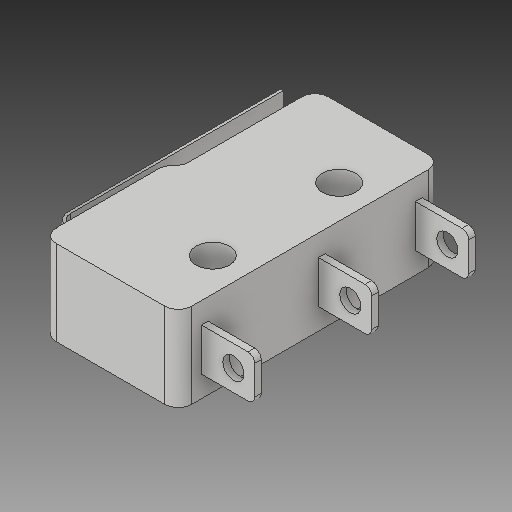
# Autodesk Inventor part: endstop_maszyna
Saved by Autodesk Inventor 2019 (Build 230136000, 136)
## iProperties
Created: 2021-11-16
Part Number: endstop_maszyna
Material: Generic
Document SubType Name: Modeling
Designer: Pokick
Density: 1 g/cm^3
Appearance: Default
Author: Pokick
Autodesk Inventor part; units mm, degrees
ref_plane "YZ Plane" through (0, 0, 0) normal (1, 0, 0) x (0, 1, 0)
ref_plane "XZ Plane" through (0, 0, 0) normal (0, 1, 0) x (-1, 0, 0)
ref_plane "XY Plane" through (0, 0, 0) normal (0, 0, 1) x (1, 0, 0)
sketch "Sketch1" plane through (0, 0, 0) normal (0, 1, 0) x (-1, 0, 0)
  line L0 (-5.1, 9.9) -> (5.1, 9.9)
  line L1 (5.1, 9.9) -> (5.1, 0.75)
  line L2 (5.1, -9.9) -> (4.4, -9.9) construction
  line L3 (-5.1, -9.9) -> (-5.1, 9.9)
  line L4 (-5.1, 9.9) -> (5.1, -9.9) construction
  line L5 (5.1, 9.9) -> (-5.1, -9.9) construction
  line L6 (0, 9.9) -> (0, 4.8) construction
  line L7 (0, 9.9) -> (5.1, 9.9) construction
  line L8 (-5.1, 4.8) -> (-2.6, 4.8) construction
  circle A0 centre (-2.6, 4.8) radius 1.25
  line L9 (-2.6, 4.8) -> (-2.6, -4.7) construction
  line L10 (-2.6, 4.8) -> (6.9, 4.8) construction
  circle A1 centre (-2.6, -4.7) radius 1.25
  line L11 (-5.1, -9.9) -> (4.4, -9.9) construction
  line L12 (-5.1, -9.9) -> (4.4, -9.9) construction
  line L13 (4.4, -9.9) -> (4.4, 0.05)
  line L14 (4.4, 0.05) -> (5.1, 0.75)
  line L15 (5.1, 0.75) -> (5.1, -9.9) construction
  line L16 (4.4, -9.9) -> (-5.1, -9.9)
  point P0 (0, 0)
  dimension "d0" = 10.2
  dimension "d1" = 19.8
  dimension "d3" = 90
  dimension "d4" = 2.5
  dimension "d5" = 5.1
  dimension "d6" = 0
  dimension "d7" = 2.5
  dimension "d8" = 9.5
  dimension "d9" = 90
  dimension "d10" = 2.5
  dimension "d11" = 9.5
  dimension "d12" = 0
  dimension "d13" = 135
  dimension "d14" = 3.0759
  constraints: 34 end point, 5 parallel, 4 horizontal, 3 equal length, 3 midpoint, 3 vertical, 2 centre point, 2 coincident, 2 collinear, 2 perpendicular, 1 point on line
  measures "d0" distance of L2.start L3.start
  measures "d1" distance of L0.end L2.start
  measures "d3" angle of L6 L7
  measures "d4" distance of L8.start L8.end
  measures "d5" distance between parallel lines of L8 L0
  measures "d6" distance from line of L7.end L1
  measures "d7" diameter of A0
  measures "d8" distance of L9.start L9.end
  measures "d9" angle of L9 L10
  measures "d10" diameter of A1
  measures "d11" distance of L3.start L11.end
  measures "d12" distance between parallel lines of L11 L12
  measures "d13" angle of L13 L14
  measures "d14" distance from line of point (0, 0) L14
extrude "Extrusion1" add sketch "Sketch1" along normal mid plane 6.4
sketch "Sketch2" plane through (0, 0, 0) normal (0, 1, 0) x (-1, 0, 0)
  line L0 (5.1, 9.9) -> (-5.1, 9.9) construction
  line L1 (-5.1, -9.9) -> (5.1, -9.9) construction
  line L2 (5.1, -9.9) -> (5.1, 9.9) construction
  line L3 (5.1, 9.9) -> (-5.1, 9.9) construction
  line L4 (-5.1, 9.9) -> (-5.1, -9.9) construction
  line L5 (-5.1, -9.9) -> (5.1, 9.9) construction
  line L6 (5.1, -9.9) -> (-5.1, 9.9) construction
  line L7 (5.1, 9.9) -> (5.1, 7.1) construction
  line L8 (5.1, 0.75) -> (5.1, 9.9) projected
  line L9 (5.1, 9.9) -> (7.9, 9.9) construction
  line L10 (5.1, 7.1) -> (7, 7.1) construction
  line L11 (5.1, 7.1) -> (7, 7.1) construction
  line L12 (7, 7.1) -> (7, -9.9) construction
  line L13 (6, 8.1) -> (8, 8.1) construction
  line L14 (8, 8.1) -> (8, 6.1) construction
  line L15 (8, 6.1) -> (6, 6.1) construction
  line L16 (6, 6.1) -> (6, 8.1) construction
  line L17 (6, 8.1) -> (8, 6.1) construction
  line L18 (8, 8.1) -> (6, 6.1) construction
  line L19 (5.1, 7.1) -> (6, 7.1)
  arc A0 (7, 6.1) -> (6, 7.1) centre (6, 6.1) ccw
  line L20 (7, 6.1) -> (7, -9.9)
  line L21 (7, -9.9) -> (6.8, -9.9)
  line L22 (6.8, -9.9) -> (6.8, 6.1)
  line L23 (5.1, 7.1) -> (5.1, 6.9)
  line L24 (5.1, 6.9) -> (6, 6.9)
  arc A1 (6.8, 6.1) -> (6, 6.9) centre (6, 6.1) ccw
  point P0 (0, 0)
  dimension "d17" = 2.8
  dimension "d18" = 90
  dimension "d19" = 1.9
  dimension "d20" = 0
  dimension "d21" = 2
  dimension "d22" = 2
  dimension "d23" = 0.2
  dimension "d24" = 90
  dimension "d25" = 0.2
  constraints: 46 end point, 6 midpoint, 5 parallel, 4 horizontal, 4 perpendicular, 4 point on circle, 4 point on line, 2 centre point, 2 collinear, 2 equal length, 2 tangent, 1 vertical
  measures "d17" distance of L0.start L7.end
  measures "d18" angle of L7 L9
  measures "d19" distance of L7.end L10.end
  measures "d20" distance between parallel lines of L10 L11
  measures "d21" distance of L14.end L15.end
  measures "d22" distance of L13.end L14.end
  measures "d23" distance of L12.end L21.end
  measures "d24" angle of L21 L8
  measures "d25" distance of L7.end L23.end
extrude "Extrusion2" add sketch "Sketch2" along normal mid plane 3.8
sketch "Sketch3" plane through (0, 0, 0) normal (0, 1, 0) x (-1, 0, 0)
  line L0 (-5.1, 9.9) -> (-5.1, -9.9) construction
  line L1 (5.1, 9.9) -> (-5.1, 9.9) construction
  line L2 (-5.1, 9.9) -> (-5.1, -9.9) construction
  line L3 (-5.1, -9.9) -> (5.1, -9.9) construction
  line L4 (5.1, -9.9) -> (5.1, 9.9) construction
  line L5 (5.1, 9.9) -> (-5.1, -9.9) construction
  line L6 (-5.1, 9.9) -> (5.1, -9.9) construction
  line L7 (-5.1, 9.9) -> (-5.1, 7.9) construction
  line L8 (-5.1, 7.9) -> (-5.1, -0.9) construction
  line L9 (-5.1, -0.9) -> (-5.1, -8.2) construction
  line L10 (-9.1, 8.15) -> (-1.1, 8.15)
  line L11 (-1.1, 8.15) -> (-1.1, 7.65)
  line L12 (-1.1, 7.65) -> (-9.1, 7.65)
  line L13 (-9.1, 7.65) -> (-9.1, 8.15)
  line L14 (-9.1, 8.15) -> (-1.1, 7.65) construction
  line L15 (-1.1, 8.15) -> (-9.1, 7.65) construction
  line L16 (-9.1, -0.65) -> (-1.1, -0.65)
  line L17 (-1.1, -0.65) -> (-1.1, -1.15)
  line L18 (-1.1, -1.15) -> (-9.1, -1.15)
  line L19 (-9.1, -1.15) -> (-9.1, -0.65)
  line L20 (-9.1, -0.65) -> (-1.1, -1.15) construction
  line L21 (-1.1, -0.65) -> (-9.1, -1.15) construction
  line L22 (-9.1, -8.45) -> (-1.1, -8.45)
  line L23 (-1.1, -8.45) -> (-1.1, -7.95)
  line L24 (-1.1, -7.95) -> (-9.1, -7.95)
  line L25 (-9.1, -7.95) -> (-9.1, -8.45)
  line L26 (-9.1, -8.45) -> (-1.1, -7.95) construction
  line L27 (-1.1, -8.45) -> (-9.1, -7.95) construction
  point P0 (0, 0)
  dimension "d28" = 2
  dimension "d29" = 8.8
  dimension "d30" = 7.3
  dimension "d31" = 8
  dimension "d32" = 0.5
  dimension "d33" = 8
  dimension "d34" = 0.5
  dimension "d35" = 8
  dimension "d36" = 0.5
  constraints: 54 end point, 8 midpoint, 8 parallel, 4 horizontal, 4 perpendicular, 3 point on line
  measures "d28" distance of L1.end L7.end
  measures "d29" distance of L7.end L8.end
  measures "d30" distance of L8.end L9.end
  measures "d31" distance of L11.end L12.end
  measures "d32" distance of L10.end L11.end
  measures "d33" distance of L17.end L18.end
  measures "d34" distance of L16.end L17.end
  measures "d35" distance of L24.end L23.end
  measures "d36" distance of L23.end L22.end
extrude "Extrusion3" add sketch "Sketch3" along normal mid plane 3.2
sketch "Sketch4" plane through (5.1, -1.6, 8.15) normal (0, 0, 1) x (1, 0, 0)
  line L0 (0, 3.2) -> (4, 3.2) construction
  line L1 (4, 0) -> (0, 0) construction
  line L2 (4, 3.2) -> (0.8, 3.2) construction
  line L3 (0.8, 3.2) -> (0.8, 0) construction
  line L4 (0.8, 0) -> (4, 0) construction
  line L5 (4, 0) -> (4, 3.2) construction
  line L6 (0.8, 3.2) -> (4, 0) construction
  line L7 (0.8, 0) -> (4, 3.2) construction
  circle A0 centre (2.4, 1.6) radius 0.8
  point P0 (-5.1, 1.6)
  dimension "d39" = 3.2
  dimension "d40" = 1.6
  constraints: 12 end point, 2 parallel, 1 centre point, 1 horizontal, 1 midpoint, 1 perpendicular, 1 point on line
  measures "d39" distance of L4.end L3.end
  measures "d40" diameter of A0
extrude "Extrusion4" cut sketch "Sketch4" against normal blind 40
fillet "Fillet1" radius 1 6 edges at (5.1, 0, 9.9) (-5.1, 0, 9.9) (-4.4, 0, -9.9) (5.1, 0, -9.9) (-4.4, 0, 0.05) (-5.1, 0, 0.75)
fillet "Fillet2" radius 0.5 6 edges at (9.1, 1.6, -8.2) (9.1, -1.6, -8.2) (9.1, -1.6, -0.9) (9.1, 1.6, -0.9) (9.1, -1.6, 7.9) (9.1, 1.6, 7.9)
body "Solid1"
